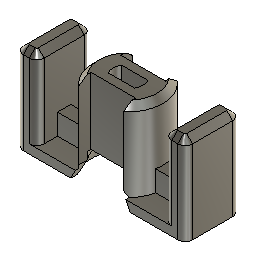
m7809_keyboard_key_shaft_v12 (Autodesk Fusion 360 design; units mm, degrees)
Autodesk Fusion 360 part; units mm, degrees
note: some values were not read from the file. Chosen so that the rebuilt part matches the saved one: which face or edge a step refers to; which pieces of a blend or face edit are solid. Set by a fixed rule: which sketch regions a step uses.
sketch "Sketch1" plane through (0, 0, 0) normal (0, 0, 1) x (1, 0, 0) in component "PLUG"
  circle A0 centre (0, 0) radius 2.35
  line L0 (-7.35, 0) -> (8.0924, 0) construction
  line L1 (0, 7.8459) -> (0, -8.5912) construction
  line L2 (-5.7, 1.85) -> (5.7, 1.85)
  line L3 (5.7, 1.85) -> (5.7, -1.85)
  line L4 (5.7, -1.85) -> (-5.7, -1.85)
  line L5 (-5.7, -1.85) -> (-5.7, 1.85)
  line L6 (-5.7, 1.85) -> (5.7, -1.85) construction
  line L7 (5.7, 1.85) -> (-5.7, -1.85) construction
  line L8 (-4.3, 1.85) -> (-4.3, -1.85)
  line L9 (4.3, 1.85) -> (4.3, -1.85)
  line L10 (1.5, 1) -> (-1.5, 1)
  line L11 (-1.5, 1) -> (-1.5, 4)
  line L12 (-1.5, 4) -> (1.5, 4)
  line L13 (1.5, 4) -> (1.5, 1)
  line L14 (1.5, 1) -> (-1.5, 4) construction
  line L15 (-1.5, 1) -> (1.5, 4) construction
  line L16 (1.5, -1) -> (-1.5, -1)
  line L17 (-1.5, -1) -> (-1.5, -4)
  line L18 (-1.5, -4) -> (1.5, -4)
  line L19 (1.5, -4) -> (1.5, -1)
  line L20 (-4.3, 0.45) -> (4.3, 0.45)
  line L21 (4.3, 0.45) -> (4.3, -0.45)
  line L22 (4.3, -0.45) -> (-4.3, -0.45)
  line L23 (-4.3, -0.45) -> (-4.3, 0.45)
  circle A1 centre (0, 0) radius 1.95
  circle A2 centre (0, 0) radius 1
  point P0 (0, 2.5)
  dimension "d1" = 4.7
  dimension "d2" = 11.4
  dimension "d3" = 3.7
  dimension "d4" = 1.4
  dimension "d5" = 3
  dimension "d6" = 3
  dimension "d7" = 2.5
  dimension "d8" = 0.9
  dimension "d9" = 0.45
  dimension "d18" = 3.9
  dimension "d23" = 2
  constraint coincident A0.centre A1.centre
  constraint horizontal L0
  constraint vertical L1
  constraint coincident A0.centre L1
  constraint coincident A0.centre L0
  constraint horizontal L2
  constraint perpendicular L2 L3
  constraint parallel L2 L4
  constraint parallel L3 L5
  constraint coincident L6 A0.centre
  constraint coincident L7 A0.centre
  constraint coincident L2 L8.start
  constraint coincident L4 L8.end
  constraint perpendicular L4 L8
  constraint symmetric L1 L8.start L9.start
  constraint symmetric L1 L8.end L9.end
  constraint horizontal L10
  constraint perpendicular L10 L11
  constraint parallel L10 L12
  constraint parallel L11 L13
  constraint coincident L14 P0
  constraint coincident L15 P0
  constraint coincident L1 P0
  constraint symmetric L0 L10.start L16.start
  constraint symmetric L0 L10.end L16.end
  constraint symmetric L0 L11.end L17.end
  constraint symmetric L0 L12.end L18.end
  constraint horizontal L20
  constraint vertical L21
  constraint horizontal L22
  constraint vertical L23
  constraint coincident L9 L21.end
  constraint coincident L8 L20.start
  constraint concentric A0 A2
  measures "d1" diameter of A0
  measures "d2" distance of L3.end L4.end
  measures "d3" distance of L2.end L3.end
  measures "d4" distance of L5 L8
  measures "d5" distance of L10.start L12.end
  measures "d6" distance of L11.end L12.end
  measures "d7" distance of L0 P0
  measures "d8" distance of L20.end L21.end
  measures "d9" distance of L0 L20
  measures "d18" diameter of A1
  measures "d23" diameter of A2
extrude "Extrude1" add sketch "Sketch1" along normal blind 0.6 contours A0 L9 L20 L21 L22 | A0 L2 L9 L13 L20 | A0 L4 L9 L19 L22 | A0 L2 L13 | A0 L4 L19 | A0 L2 L11 | A0 L4 L17 | A0 L2 L8 L11 L20 | A0 L4 L8 L17 L22 | A0 L8 L20 L22 L23 makes body 1 at (3.6481, -0.0546, 0.6) makes body 2 at (-3.6481, -0.0546, 0) in component "PLUG"
extrude "Extrude2" add sketch "Sketch1" along normal blind 6 contours A0 L20 L22 A1 | A0 L13 L20 A1 | A0 L19 L22 A1 | L20 L22 A1 A2 | L10 L13 L20 A1 A2 | L16 L19 L22 A1 A2 | L20 L22 A2 | L20 A2 | L22 A2 | L20 L22 A1 A2 | L10 L11 L20 A1 A2 | L16 L17 L22 A1 A2 | A0 L11 L20 A1 | A0 L20 L22 A1 | A0 L17 L22 A1 bodies 1 2 in component "PLUG"
extrude "Extrude3" add sketch "Sketch1" along normal blind 6 contours L2 L3 L4 L9 L21 | L2 L4 L5 L8 L23 bodies 1 in component "PLUG"
fillet "Fillet1" radius 0.5 8 edges at (5.7, -1.85, 3) (5.7, 1.85, 3) (-5.7, -1.85, 3) (-5.7, 1.85, 3) (-4.3, 1.85, 3.3) (-4.3, -1.85, 3.3) (4.3, 1.85, 3.3) (4.3, -1.85, 3.3) on bodies 1 in component "PLUG"
extrude "Extrude4" cut sketch "Sketch1" along normal blind 1.5 contours A0 L2 L13 A1 | A0 L2 L13 | L20 L22 A1 A2 | L10 L13 L20 A1 A2 | A0 L4 L19 | A0 L4 L19 A1 | L16 L19 L22 A1 A2 | A0 L2 A1 | A0 L2 L11 L12 L13 | L2 L10 L11 L13 A1 | L20 L22 A2 | L20 A2 | A0 L4 L17 L18 L19 | A0 L4 A1 | L4 L16 L17 L19 A1 | L22 A2 | A0 L2 L11 A1 | A0 L2 L11 | L2 A1 | L20 L22 A1 A2 | L10 L11 L20 A1 A2 | A0 L4 L17 | A0 L4 L17 A1 | L4 A1 | L16 L17 L22 A1 A2 bodies 1 in component "PLUG"
extrude "Extrude5" add sketch "Sketch1" along normal blind 2 contours A0 L9 L20 L21 L22 | A0 L8 L20 L22 L23 bodies 1 in component "PLUG"
extrude "Extrude6" cut sketch "Sketch1" along normal through all contours L20 L22 A2 bodies 1 in component "PLUG"
chamfer "Chamfer1" distance 0.4 angle 45 18 edges at (-2.35, 0, 6) (2.35, 0, 6) (4.3, 0, 6) (4.4464, -1.7036, 6) (5, -1.85, 6) (5.5536, -1.7036, 6) (5.7, 0, 6) (5.5536, 1.7036, 6) (5, 1.85, 6) (4.4464, 1.7036, 6) (-4.3, 0, 6) (-4.4464, 1.7036, 6) (-5, 1.85, 6) (-5.5536, 1.7036, 6) (-5.7, 0, 6) (-5.5536, -1.7036, 6) (-5, -1.85, 6) (-4.4464, -1.7036, 6) on bodies 1 in component "PLUG"
chamfer "Chamfer2" distance 0.5 distance2 1 6 edges at (1.95, 0, 0) (-1.95, 0, 0) (-1.5, -1.548, 0) (1.5, -1.548, 0) (1.5, 1.548, 0) (-1.5, 1.548, 0) measured on face at (4.45, 0, 0) measured on face at (-4.45, 0, 0) measured on face at (-4.45, 0, 0) measured on face at (4.45, 0, 0) measured on face at (4.45, 0, 0) measured on face at (-1.5, 1.2697, 4.3667) on bodies 1 in component "PLUG"
component "PLUG" placed x (1, 0, 0) y (0, 1, 0) z (0, 0, 1) at (0, 0, 0)
equation "d9 = d8 / 2"
